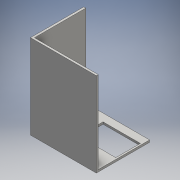
# Autodesk Inventor part: RoomEnvironment
Saved by Autodesk Inventor 2016 (Build 200138000, 138)
## iProperties
Created: 2015-11-22
Part Number: RoomEnvironment
Material: 常规
Document SubType Name: Modeling
Designer: Shawn Shi Feng
Density: 1 g/cm^3
Appearance: 默认
Author: Shawn Shi Feng
Autodesk Inventor part; units mm, degrees
ref_plane "YZ Plane" through (0, 0, 0) normal (1, 0, 0) x (0, 1, 0)
ref_plane "XZ Plane" through (0, 0, 0) normal (0, 1, 0) x (-1, 0, 0)
ref_plane "XY Plane" through (0, 0, 0) normal (0, 0, 1) x (1, 0, 0)
sketch "草图1" plane through (0, 0, 0) normal (0, 0, 1) x (1, 0, 0)
  line L0 (-2968.4868, 2431.0636) -> (156.5132, 2431.0636)
  line L1 (156.5132, 2431.0636) -> (156.5132, -93.9364)
  line L2 (156.5132, -93.9364) -> (-2968.4868, -93.9364)
  line L3 (-2968.4868, -93.9364) -> (-2968.4868, 2431.0636)
  line L4 (-1688.4868, 2071.0636) -> (81.5132, 2071.0636)
  line L5 (81.5132, 2071.0636) -> (81.5132, 901.0636)
  line L6 (81.5132, 901.0636) -> (-1688.4868, 901.0636)
  line L7 (-1688.4868, 901.0636) -> (-1688.4868, 2071.0636)
  line L8 (-2968.4868, 2188.5636) -> (-2968.4868, 2431.0636)
  line L9 (-2968.4868, -93.9364) -> (156.5132, -93.9364)
  line L10 (156.5132, -93.9364) -> (156.5132, -83.9364)
  line L11 (-2968.4868, -83.9364) -> (-2968.4868, -93.9364)
  point P0 (0, 0)
  dimension "d0" = 3125
  dimension "d1" = 2525
  dimension "d2" = 360
  dimension "d3" = 75
  dimension "d4" = 1770
  dimension "d5" = 1170
  constraints: 24 end point, 5 parallel, 3 horizontal, 3 perpendicular, 1 point on line
  measures "d0" distance of L1.end L2.end
  measures "d1" distance of L0.end L1.end
  measures "d2" distance between parallel lines of L4 L0
  measures "d3" distance between parallel lines of L1 L5
  measures "d4" distance of L5.end L6.end
  measures "d5" distance of L4.end L5.end
extrude "拉伸1" add sketch "草图1" against normal blind 100
sketch "草图3" plane through (0, 0, 0) normal (0, 0, 1) x (1, 0, 0)
  line L0 (-2968.4868, 2431.0636) -> (156.5132, 2431.0636) projected
  line L1 (-2868.4868, 2431.0636) -> (-2968.4868, 2431.0636)
  line L2 (-2968.4868, 2431.0636) -> (-2968.4868, -93.9364)
  line L3 (-2968.4868, -93.9364) -> (-2868.4868, -93.9364)
  line L4 (-2868.4868, -93.9364) -> (-2868.4868, 2431.0636)
  point P0 (0, 0)
  dimension "d16" = 100
  constraints: 8 end point, 2 parallel, 1 horizontal, 1 perpendicular, 1 point on line
  measures "d16" distance between parallel lines of L4 L2
extrude "拉伸2" add sketch "草图3" along normal blind 3900
sketch "草图4" plane through (0, 0, 0) normal (0, 0, 1) x (1, 0, 0)
  line L0 (-2868.4868, 2431.0636) -> (-2868.4868, -93.9364) projected
  line L1 (156.5132, -93.9364) -> (-2868.4868, -93.9364)
  line L2 (-2868.4868, -93.9364) -> (-2868.4868, 0)
  line L3 (-2868.4868, 0) -> (156.5132, 0)
  line L4 (156.5132, 0) -> (156.5132, -93.9364)
  point P0 (0, 0)
  constraints: 8 end point, 2 parallel, 1 horizontal, 1 perpendicular, 1 point on line
extrude "拉伸3" add sketch "草图4" along normal blind 3900
